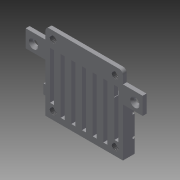
# Autodesk Inventor part: LensBaseTop01
Saved by Autodesk Inventor 2015 (Build 190159000, 159)
## iProperties
Created: 2014-07-30
Part Number: LensBaseTop01
Material: Generic
Document SubType Name: Modeling
Designer: spichelh
Density: 1 g/cm^3
Appearance: Default
Author: spichelh
Autodesk Inventor part; units mm, degrees
ref_plane "YZ Plane" through (0, 0, 0) normal (1, 0, 0) x (0, 1, 0)
ref_plane "XZ Plane" through (0, 0, 0) normal (0, 1, 0) x (-1, 0, 0)
ref_plane "XY Plane" through (0, 0, 0) normal (0, 0, 1) x (1, 0, 0)
sketch "Sketch1" plane through (0, 0, 0) normal (0, 0, 1) x (1, 0, 0)
  circle A0 centre (56.34, 4) radius 1.4
  circle A1 centre (4, 4) radius 1.4
  line L0 (16.17, 3) -> (19.17, 3)
  line L1 (19.17, 3) -> (19.17, 7)
  line L2 (19.17, 7) -> (21.17, 7)
  line L3 (21.17, 7) -> (21.17, 3)
  line L4 (21.17, 3) -> (24.17, 3)
  line L5 (24.17, 3) -> (24.17, 7)
  line L6 (24.17, 7) -> (26.17, 7)
  line L7 (26.17, 7) -> (26.17, 3)
  line L8 (26.17, 3) -> (29.17, 3)
  line L9 (29.17, 3) -> (29.17, 7)
  line L10 (29.17, 7) -> (31.17, 7)
  line L11 (31.17, 7) -> (31.17, 3)
  line L12 (31.17, 3) -> (34.17, 3)
  line L13 (34.17, 3) -> (34.17, 7)
  line L14 (34.17, 7) -> (36.17, 7)
  line L15 (36.17, 7) -> (36.17, 3)
  line L16 (36.17, 3) -> (39.17, 3)
  line L17 (39.17, 3) -> (39.17, 7)
  line L18 (39.17, 7) -> (41.17, 7)
  line L19 (41.17, 7) -> (41.17, 3)
  line L20 (41.17, 3) -> (44.17, 3)
  line L21 (44.17, 3) -> (44.17, 7)
  line L22 (44.17, 7) -> (46.17, 7)
  line L23 (46.17, 7) -> (46.17, 3)
  line L24 (46.17, 3) -> (50.17, 3)
  line L25 (50.17, 3) -> (50.17, 0)
  line L26 (50.17, 0) -> (60.34, 0)
  line L27 (60.34, 0) -> (60.34, 9)
  line L28 (0, 9) -> (60.34, 9)
  line L29 (0, 0) -> (0, 9)
  line L30 (0, 0) -> (10.17, 0)
  line L31 (10.17, 0) -> (10.17, 3)
  line L32 (10.17, 3) -> (14.17, 3)
  line L33 (14.17, 3) -> (14.17, 7)
  line L34 (14.17, 7) -> (16.17, 7)
  line L35 (16.17, 7) -> (16.17, 3)
  line L36 (60.34, 9) -> (60.34, 17.91156)
  line L37 (50.17, -25) -> (10.17, -25)
  line L38 (0, 0) -> (0, 9)
  line L39 (10.17, -25) -> (50.17, -25) construction
  line L40 (50.17, -25) -> (50.17, 15) construction
  line L41 (50.17, 15) -> (10.17, 15) construction
  line L42 (10.17, 15) -> (10.17, -25) construction
  line L43 (30.17, 15) -> (30.17, 11.566651) construction
  line L44 (30.17, -25) -> (30.17, -12.329025) construction
  circle A2 centre (14.17, -21) radius 1.75
  line L45 (50.17, -5) -> (45.17, -5) construction
  circle A3 centre (46.17, -21) radius 1.75
  circle A4 centre (14.17, 11) radius 1.75
  circle A5 centre (46.17, 11) radius 1.75
  line L46 (0, 0) -> (10.17, 0)
  line L47 (10.17, 0) -> (10.17, -25)
  line L48 (60.34, 17.91156) -> (50.17, 17.91156)
  line L49 (50.17, 0) -> (50.17, -25)
  line L50 (10.17, 15) -> (10.17, 9)
  line L51 (50.17, 15) -> (50.17, 9)
  line L52 (50.17, 9) -> (60.34, 9)
  line L53 (10.17, 9) -> (0, 9)
  line L54 (10.17, 15) -> (50.17, 15)
  dimension "d10" = 40
  dimension "d11" = 40
  dimension "d12" = 3.5
  dimension "d46" = 32
  dimension "d47" = 32
  dimension "d48" = 6
  constraints: 36 end point, 9 collinear, 7 point on line, 4 centre point, 4 parallel, 3 midpoint, 3 symmetric about line, 2 perpendicular, 1 horizontal, 5 other
  measures "d10" distance of L41.end L40.end
  measures "d11" distance between parallel lines of L39 L41
  measures "d12" diameter of A2
  measures "d46" distance of A5.centre A4.centre
  measures "d47" distance of A5.centre A3.centre
  measures "d48" distance between parallel lines of L28 L54
extrude "Extrusion1" add sketch "Sketch1" along normal blind 2
sketch "Sketch2" plane through (0, 0, 0) normal (0, 0, -1) x (-1, 0, 0)
  line L0 (-50.17, -25) -> (-10.17, -25)
  line L1 (-10.17, -25) -> (-10.17, -18)
  line L2 (-10.17, -18) -> (-50.17, -18)
  line L3 (-50.17, -18) -> (-50.17, -25)
  circle A0 centre (-46.17, -21) radius 1.75 projected
  circle A1 centre (-14.17, -21) radius 1.75 projected
  circle A2 centre (-4, 4) radius 1.4 projected
  circle A3 centre (-56.34, 4) radius 1.4 projected
  line L4 (0, 0) -> (-10.17, 0) projected
  line L5 (-50.17, 0) -> (-60.34, 0) projected
  line L6 (-50.17, -25) -> (-50.17, 0) projected
  line L7 (-10.17, -25) -> (-50.17, -25) projected
  line L8 (-10.17, 0) -> (-10.17, -25) projected
  line L9 (-50.17, -25) -> (-50.17, 0) projected
  line L10 (-10.17, 0) -> (-10.17, -25) projected
  line L11 (-50.17, -17) -> (-10.17, -17)
  line L12 (-10.17, -17) -> (-10.17, -7)
  line L13 (-10.17, -7) -> (-50.17, -7)
  line L14 (-50.17, -7) -> (-50.17, -17)
  line L15 (-50.17, -6) -> (-10.17, -6)
  line L16 (-10.17, -6) -> (-10.17, -1)
  line L17 (-10.17, -1) -> (-50.17, -1)
  line L18 (-50.17, -1) -> (-50.17, -6)
  line L19 (-60.34, 9) -> (-50.17, 9) projected
  line L20 (-50.17, 15) -> (-10.17, 15) projected
  line L21 (-50.17, 9) -> (-50.17, 15) projected
  line L22 (-10.17, 15) -> (-10.17, 9) projected
  line L23 (-60.34, 0) -> (-60.34, 9) projected
  line L24 (0, 9) -> (0, 0) projected
  line L25 (-10.17, 9) -> (0, 9) projected
  dimension "d16" = 7
  dimension "d18" = 1
  dimension "d19" = 10
  dimension "d31" = 1
  dimension "d32" = 5
  constraints: 24 end point, 6 parallel, 4 point on line, 3 collinear, 3 horizontal, 3 perpendicular
  measures "d16" distance between parallel lines of L0 L2
  measures "d18" distance between parallel lines of L2 L11
  measures "d19" distance between parallel lines of L13 L11
  measures "d31" distance between parallel lines of L13 L15
  measures "d32" distance between parallel lines of L17 L15
extrude "Extrusion2" add sketch "Sketch2" along normal blind 4 contours L3 L2 L1 L0 | L6 L13 L8 L11 | L6 L17 L8 L15 | A0 | A1
sketch "Sketch3" plane through (0, 0, 0) normal (0, 0, -1) x (-1, 0, 0)
  line L0 (-50.17, -18) -> (-10.17, -18) projected
  line L1 (-10.17, -17) -> (-10.17, -25) projected
  line L2 (-10.17, -17) -> (-50.17, -17) projected
  line L3 (-50.17, -25) -> (-50.17, -17) projected
  line L4 (-10.17, 0) -> (-10.17, -1) projected
  line L5 (-50.17, -1) -> (-50.17, 0) projected
  line L6 (-50.17, -18) -> (-50.17, -17) projected
  line L7 (-10.17, -17) -> (-10.17, -18) projected
  line L8 (0, 0) -> (-10.17, 0) projected
  line L9 (-50.17, 0) -> (-60.34, 0) projected
  line L10 (0, 0) -> (-10.17, 0) projected
  line L11 (-50.17, 0) -> (-60.34, 0) projected
  line L12 (-50.17, -1) -> (-10.17, -1) projected
  line L13 (-10.17, 0) -> (-10.17, -1) projected
  line L14 (-50.17, -1) -> (-50.17, 0) projected
  line L15 (-50.17, -18) -> (-10.17, -18) projected
  line L16 (-10.17, -17) -> (-50.17, -17) projected
  line L17 (-50.17, -1) -> (-10.17, -1) projected
  line L18 (-50.17, -18) -> (-10.17, -18) projected
  line L19 (-10.17, -17) -> (-10.17, -18) projected
  line L20 (-10.17, -17) -> (-50.17, -17) projected
  line L21 (-50.17, -18) -> (-50.17, -17) projected
  line L22 (-10.17, -6) -> (-50.17, -6) projected
  line L23 (-50.17, -7) -> (-50.17, -6) projected
  line L24 (-50.17, -7) -> (-10.17, -7) projected
  line L25 (-10.17, -6) -> (-10.17, -7) projected
  line L26 (-50.17, 0) -> (-10.17, 0)
  line L27 (-10.17, 0) -> (-10.17, -1)
  line L28 (-10.17, -1) -> (-50.17, -1)
  line L29 (-50.17, -1) -> (-50.17, 0)
  line L30 (-60.34, 9) -> (-50.17, 9) projected
  line L31 (-60.34, 9) -> (-50.17, 9) projected
  line L32 (-10.17, 15) -> (-10.17, 9) projected
  line L33 (-50.17, 15) -> (-10.17, 15) projected
  line L34 (-50.17, 9) -> (-50.17, 15) projected
  line L35 (-10.17, 15) -> (-10.17, 9) projected
  line L36 (-50.17, 15) -> (-10.17, 15) projected
  line L37 (-50.17, 9) -> (-50.17, 15) projected
  line L38 (0, 9) -> (0, 0) projected
  line L39 (-10.17, 9) -> (0, 9) projected
  line L40 (-60.34, 0) -> (-60.34, 9) projected
  line L41 (0, 9) -> (0, 0) projected
  line L42 (-10.17, 9) -> (0, 9) projected
  line L43 (-60.34, 0) -> (-60.34, 9) projected
  constraints: 8 end point, 2 parallel, 1 horizontal, 1 perpendicular
extrude "Extrusion3" add sketch "Sketch3" along normal blind 3 contours L3 L2 L1 L0 | L4 L12 L5 L26 | L25 L24 L23 L22
sketch "Sketch5" plane through (10.17, -25, 2) normal (-1, 0, 0) x (0, 0, 1)
  line L0 (-6, 8) -> (-6, 18) projected
  line L1 (-5, 8) -> (-6, 8) projected
  line L2 (-6, 7) -> (-6, 8) projected
  line L3 (-5, 7) -> (-6, 7) projected
  line L4 (-6, 0) -> (-6, 7) projected
  line L5 (0, 25) -> (0, 0) projected
  line L6 (-6, 10) -> (0, 10)
  line L7 (-6, 5) -> (0, 5)
  line L8 (-4, 10) -> (-4, 5)
  point P0 (-3, 8)
  point P1 (-3, 7)
  dimension "d25" = 2
  dimension "d26" = 2
  dimension "d27" = 2
  constraints: 6 end point, 6 point on line, 3 perpendicular
  measures "d25" distance between parallel lines of L6 L1
  measures "d26" distance between parallel lines of L7 L3
  measures "d27" distance between parallel lines of L8 L2
sketch "Sketch5 outline for Extrusion4" plane through (10.17, -25, 2) normal (-1, 0, 0) x (0, 0, 1)
  line L0 (-6, 10) -> (-6, 8)
  line L1 (-4, 10) -> (-6, 10)
  line L2 (-4, 5) -> (-4, 10)
  line L3 (-6, 5) -> (-4, 5)
  line L4 (-6, 7) -> (-6, 5)
  line L5 (-5, 7) -> (-6, 7)
  line L6 (-5, 8) -> (-5, 7)
  line L7 (-6, 8) -> (-5, 8)
extrude "Extrusion4" add sketch "Sketch5 outline for Extrusion4" along normal blind 5
chamfer "Chamfer1" distance 1 angle 45 2 edges at (2.6, 4, 2) (54.94, 4, 2)
thread "Thread1" size "M3x0.5" class "6H" standard "ANSI Metric M Profile" full length
thread "Thread2" size "M3x0.5" class "6H" standard "ANSI Metric M Profile" full length
thread "Thread3" size "M3x0.5" class "6H" standard "ANSI Metric M Profile" full length
thread "Thread4" size "M3x0.5" class "6H" standard "ANSI Metric M Profile" full length
sketch "Sketch6" plane through (0, 0, 2) normal (0, 0, 1) x (1, 0, 0)
  line L0 (20.035459, 6.5) -> (20.035459, 1)
  line L1 (20.035459, 1) -> (18.035459, 1)
  line L2 (18.035459, 1) -> (18.035459, 6.5)
  line L3 (18.035459, 6.5) -> (20.035459, 6.5)
  line L4 (31.035459, 6.5) -> (31.035459, 1)
  line L5 (31.035459, 1) -> (29.035459, 1)
  line L6 (29.035459, 1) -> (29.035459, 6.5)
  line L7 (29.035459, 6.5) -> (31.035459, 6.5)
  line L8 (42.035459, 6.5) -> (42.035459, 1)
  line L9 (42.035459, 1) -> (40.035459, 1)
  line L10 (40.035459, 1) -> (40.035459, 6.5)
  line L11 (40.035459, 6.5) -> (42.035459, 6.5)
  line L12 (47.535459, 6.5) -> (47.535459, 1)
  line L13 (47.535459, 1) -> (45.535459, 1)
  line L14 (45.535459, 1) -> (45.535459, 6.5)
  line L15 (45.535459, 6.5) -> (47.535459, 6.5)
  line L16 (36.535459, 6.5) -> (36.535459, 1)
  line L17 (36.535459, 1) -> (34.535459, 1)
  line L18 (34.535459, 1) -> (34.535459, 6.5)
  line L19 (34.535459, 6.5) -> (36.535459, 6.5)
  line L20 (25.535459, 6.5) -> (25.535459, 1)
  line L21 (25.535459, 1) -> (23.535459, 1)
  line L22 (23.535459, 1) -> (23.535459, 6.5)
  line L23 (23.535459, 6.5) -> (25.535459, 6.5)
  line L24 (14.535459, 6.5) -> (14.535459, 1)
  line L25 (14.535459, 1) -> (12.535459, 1)
  line L26 (12.535459, 1) -> (12.535459, 6.5)
  line L27 (12.535459, 6.5) -> (14.535459, 6.5)
  line L28 (6.600091, -5) -> (0.399703, -5)
  line L29 (53.739909, -5) -> (53.739909, 0)
  line L30 (52.54, 0) -> (53.739909, 0)
  line L31 (52.54, 0) -> (52.54, 1)
  line L32 (52.54, 1) -> (51.035459, 1)
  line L33 (51.035459, 1) -> (51.035459, 6.5)
  line L34 (51.035459, 6.5) -> (52.54, 6.5)
  line L35 (52.54, 6.5) -> (52.54, 7)
  line L36 (52.54, 7) -> (7.8, 7)
  line L37 (7.8, 6.5) -> (7.8, 7)
  line L38 (7.8, 6.5) -> (9.035459, 6.5)
  line L39 (9.035459, 6.5) -> (9.035459, 1)
  line L40 (9.035459, 1) -> (7.8, 1)
  line L41 (7.8, 0) -> (7.8, 1)
  line L42 (6.600091, 0) -> (7.8, 0)
  line L43 (6.600091, 0) -> (6.600091, -5)
  line L44 (59.940297, -5) -> (53.739909, -5)
  line L45 (7.8, -6) -> (7.8, -5)
  line L46 (52.54, -5) -> (7.8, -5)
  line L47 (52.54, -5) -> (52.54, -6)
  line L48 (10.17, -25) -> (50.17, -25)
  line L49 (12.535459, 6.5) -> (14.535459, 6.5)
  line L50 (14.535459, 6.5) -> (14.535459, -18)
  line L51 (14.535459, -18) -> (12.535459, -18)
  line L52 (12.535459, -18) -> (12.535459, 6.5)
  line L53 (30.17, -25) -> (30.17, -17.216661) construction
  line L54 (47.804541, 6.5) -> (45.804541, 6.5)
  line L55 (45.804541, 6.5) -> (45.804541, -18)
  line L56 (45.804541, -18) -> (47.804541, -18)
  line L57 (47.804541, -18) -> (47.804541, 6.5)
  line L58 (18.035459, 6.5) -> (20.035459, 6.5)
  line L59 (20.035459, 6.5) -> (20.035459, -22)
  line L60 (20.035459, -22) -> (18.035459, -22)
  line L61 (18.035459, -22) -> (18.035459, 6.5)
  line L62 (23.535459, 6.5) -> (25.535459, 6.5)
  line L63 (25.535459, 6.5) -> (25.535459, -22)
  line L64 (25.535459, -22) -> (23.535459, -22)
  line L65 (23.535459, -22) -> (23.535459, 6.5)
  line L66 (29.035459, 6.5) -> (31.035459, 6.5)
  line L67 (31.035459, 6.5) -> (31.035459, -22)
  line L68 (31.035459, -22) -> (29.035459, -22)
  line L69 (29.035459, -22) -> (29.035459, 6.5)
  line L70 (34.535459, 6.5) -> (36.535459, 6.5)
  line L71 (36.535459, 6.5) -> (36.535459, -22)
  line L72 (36.535459, -22) -> (34.535459, -22)
  line L73 (34.535459, -22) -> (34.535459, 6.5)
  line L74 (40.035459, 6.5) -> (42.035459, 6.5)
  line L75 (42.035459, 6.5) -> (42.035459, -22)
  line L76 (42.035459, -22) -> (40.035459, -22)
  line L77 (40.035459, -22) -> (40.035459, 6.5)
  line L78 (52.54, -6) -> (60.34, -6)
  line L79 (60.34, 0) -> (60.34, -6)
  line L80 (59.940297, 0) -> (60.34, 0)
  line L81 (59.940297, 0) -> (59.940297, -5)
  line L82 (0.399703, -5) -> (0.399703, 0)
  line L83 (0, 0) -> (0.399703, 0)
  line L84 (0, 0) -> (0, -6)
  line L85 (0, -6) -> (7.8, -6)
  dimension "d51" = 7
  dimension "d53" = 3
  dimension "d56" = 5.5
  constraints: 58 end point, 6 collinear, 4 parallel, 4 symmetric about line, 3 horizontal, 3 perpendicular, 1 midpoint, 32 other
  measures "d51" distance between parallel lines of L48 L51
  measures "d53" distance between parallel lines of L48 L60
  measures "d56" distance of L59.end L64.start
sketch "Sketch6 outline for Extrusion5" plane through (0, 0, 2) normal (0, 0, 1) x (1, 0, 0)
  line L0 (12.535459, 6.5) -> (14.535459, 6.5)
  line L1 (12.535459, 6.5) -> (12.535459, -18)
  line L2 (14.535459, -18) -> (12.535459, -18)
  line L3 (14.535459, -18) -> (14.535459, 6.5)
  line L4 (45.535459, 1) -> (45.535459, 6.5)
  line L5 (45.804541, 1) -> (45.535459, 1)
  line L6 (45.804541, -18) -> (45.804541, 1)
  line L7 (47.804541, -18) -> (45.804541, -18)
  line L8 (47.804541, 6.5) -> (47.804541, -18)
  line L9 (47.804541, 6.5) -> (45.535459, 6.5)
  line L10 (18.035459, 6.5) -> (20.035459, 6.5)
  line L11 (18.035459, 6.5) -> (18.035459, -22)
  line L12 (20.035459, -22) -> (18.035459, -22)
  line L13 (20.035459, -22) -> (20.035459, 6.5)
  line L14 (23.535459, -22) -> (25.535459, -22)
  line L15 (25.535459, -22) -> (25.535459, 6.5)
  line L16 (25.535459, 6.5) -> (23.535459, 6.5)
  line L17 (23.535459, 6.5) -> (23.535459, -22)
  line L18 (29.035459, -22) -> (31.035459, -22)
  line L19 (31.035459, -22) -> (31.035459, 6.5)
  line L20 (31.035459, 6.5) -> (29.035459, 6.5)
  line L21 (29.035459, 6.5) -> (29.035459, -22)
  line L22 (34.535459, -22) -> (36.535459, -22)
  line L23 (36.535459, -22) -> (36.535459, 6.5)
  line L24 (36.535459, 6.5) -> (34.535459, 6.5)
  line L25 (34.535459, 6.5) -> (34.535459, -22)
  line L26 (40.035459, -22) -> (42.035459, -22)
  line L27 (42.035459, -22) -> (42.035459, 6.5)
  line L28 (42.035459, 6.5) -> (40.035459, 6.5)
  line L29 (40.035459, 6.5) -> (40.035459, -22)
extrude "Extrusion5" cut sketch "Sketch6 outline for Extrusion5" against normal blind 8
fillet "Fillet1" radius 2 2 edges at (10.17, 15, 1) (50.17, 15, 1)
body "Solid1"
